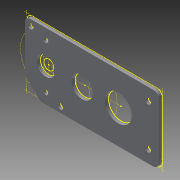
# Autodesk Inventor part: Granny Gearbox Input Plate Routing Template
Saved by Autodesk Inventor 2015 (Build 190159000, 159)
## iProperties
Created: 2016-02-25
Part Number: Granny Gearbox Input Plate Routing Template
Material: Generic
Document SubType Name: Modeling
Designer: sethbattis
Density: 1 g/cm^3
Appearance: Default
Author: sethbattis
Autodesk Inventor part; units mm, degrees
ref_plane "YZ Plane" through (0, 0, 0) normal (1, 0, 0) x (0, 1, 0)
ref_plane "XZ Plane" through (0, 0, 0) normal (0, 1, 0) x (-1, 0, 0)
ref_plane "XY Plane" through (0, 0, 0) normal (0, 0, 1) x (1, 0, 0)
derived "Granny Gearbox Input Plate.ipt"
feature "Solid1::Granny Gearbox Input Plate.ipt" [suppressed]
sketch "Shaft Alignment" plane through (0, 0, 0) normal (0, 0, 1) x (1, 0, 0)
  line L0 (-40.7035, -5.5985) -> (-0.0001, -11.1125) construction
  line L1 (-35.1409, -0.031) -> (-35.1353, -6.3528) construction
  line L2 (-11.1125, -0.0098) -> (-11.104, -9.6083) construction
  line L3 (0, 11.1125) -> (43.74, 13.9583) construction
  line L4 (-40.7035, -5.5985) -> (-46.2661, -5.5985) construction
  line L5 (-40.7035, -19.8733) -> (-46.2661, -19.8733) construction
  line L6 (-40.7035, 19.8015) -> (-46.2661, 19.8015) construction
  line L7 (-40.7035, 5.5267) -> (-46.2661, 5.5267) construction
  line L8 (-46.2661, 25.3641) -> (-46.2661, -25.4359) construction
  line L9 (-40.7035, 25.3641) -> (-40.7035, -25.4359) construction
  line L10 (-40.7035, -0.0359) -> (0, 0) construction
  line L11 (0, 0) -> (40.6908, 0) construction
  line L12 (11.1125, 0) -> (11.1125, 11.8355) construction
  line L13 (26.4033, 0) -> (26.4033, 12.8304) construction
  circle A0 centre (-40.7035, 25.3641) radius 5.5626
  circle A1 centre (-40.7035, -25.4359) radius 5.5626
  circle A2 centre (40.6908, 0) radius 14.2875
  circle A3 centre (0, 0) radius 11.1125
  circle A4 centre (-40.7035, -0.0359) radius 5.5626
  point P0 (-33.5787, -27.5177)
sketch "New Mounting Holes" plane through (0, 0, 0) normal (0, 0, 1) x (1, 0, 0)
  circle A0 centre (-40.7035, -0.0359) radius 31.75 construction
  circle A1 centre (40.6908, 0) radius 36.195 construction
  circle A2 centre (0, 0) radius 36.195 construction
  line L0 (-57.7242, 30.4609) -> (-55.8383, 30.4609) construction
  line L1 (-57.7242, 30.4609) -> (-57.7242, 28.575) construction
  circle A3 centre (-57.7242, 30.4609) radius 3.175
  circle A4 centre (-24.3812, -30.912) radius 3.175
  line L2 (-65.3633, -38.1) -> (-65.3633, 38.1) construction
  line L3 (87.0367, -38.1) -> (-65.3633, -38.1) construction
  line L4 (87.0367, 38.1) -> (87.0367, -38.1) construction
  line L5 (-65.3633, 38.1) -> (87.0367, 38.1) construction
  line L6 (-55.8383, 38.1) -> (-55.8383, -38.1) construction
  line L7 (-65.3633, 28.575) -> (87.0367, 28.575) construction
  line L8 (-65.3633, -28.575) -> (87.0367, -28.575) construction
  line L9 (77.5117, 38.1) -> (77.5117, -38.1) construction
  circle A5 centre (74.3367, 23.3553) radius 3.175
  circle A6 centre (74.3367, -23.3553) radius 3.175
sketch "Labels" plane through (0, 0, 0) normal (0, 0, 1) x (1, 0, 0)
  circle A0 centre (-40.7035, -0.0359) radius 5.5626
  circle A1 centre (-40.7035, 25.3641) radius 5.5626
  circle A2 centre (-40.7035, -25.4359) radius 5.5626
  circle A3 centre (0, 0) radius 11.1125
  circle A4 centre (40.6908, 0) radius 14.2875
  line L0 (-5.8677, 26.2224) -> (48.5566, 26.2224) construction
  line L1 (48.5566, 26.2224) -> (48.5566, 22.1963) construction
  line L2 (48.5566, 22.1963) -> (-5.8677, 22.1963) construction
  line L3 (-5.8677, 22.1963) -> (-5.8677, 26.2224) construction
sketch "Exterior" plane through (0, 0, 0) normal (0, 0, 1) x (1, 0, 0)
  line L0 (-65.3633, -17.4045) -> (-65.3633, 31.75)
  line L1 (-59.0133, 38.1) -> (80.6867, 38.1)
  line L2 (87.0367, 31.75) -> (87.0367, -31.75)
  line L3 (80.6867, -38.1) -> (-44.6678, -38.1)
  arc A0 (87.0367, 31.75) -> (80.6867, 38.1) centre (80.6867, 31.75) ccw
  arc A1 (80.6867, -38.1) -> (87.0367, -31.75) centre (80.6867, -31.75) ccw
  arc A2 (-59.0133, 38.1) -> (-65.3633, 31.75) centre (-59.0133, 31.75) ccw
  circle A3 centre (-40.7035, -0.0359) radius 31.75 construction
  line L4 (-63.5034, -21.8946) -> (-49.1579, -36.2401)
  line L5 (-65.3633, -38.1) -> (-65.3633, 38.1) construction
  line L6 (87.0367, -38.1) -> (-65.3633, -38.1) construction
  arc A4 (-49.1579, -36.2401) -> (-44.6678, -38.1) centre (-44.6678, -31.75) ccw
  arc A5 (-65.3633, -17.4045) -> (-63.5034, -21.8946) centre (-59.0133, -17.4045) ccw
  point P0 (87.0367, 38.1)
  point P1 (-65.3633, -20.0348)
  point P2 (-47.2981, -38.1)
sketch "Input Labels" plane through (0, 0, 0) normal (0, 0, 1) x (1, 0, 0)
  circle A0 centre (-40.7035, 25.3641) radius 2.667
  circle A1 centre (-40.7035, -0.0359) radius 9.525
  circle A2 centre (-40.7035, -25.4359) radius 2.667
  circle A3 centre (0, 0) radius 11.1125
  line L0 (-5.8677, 22.1963) -> (-5.8677, 26.2224) construction
  line L1 (-5.8677, 26.2224) -> (48.5566, 26.2224) construction
  line L2 (48.5566, 26.2224) -> (48.5566, 22.1963) construction
  line L3 (48.5566, 22.1963) -> (-5.8677, 22.1963) construction
  circle A4 centre (40.6908, 0) radius 14.2875
  line L4 (-5.8677, 26.2224) -> (45.7507, 26.2224) construction
  line L5 (45.7507, 26.2224) -> (45.7507, 22.1963) construction
  line L6 (45.7507, 22.1963) -> (-5.8677, 22.1963) construction
  line L7 (-5.8677, 22.1963) -> (-5.8677, 26.2224) construction
sketch "Sketch6" plane through (0, 0, 0) normal (0, 0, 1) x (1, 0, 0)
  line L0 (-63.5034, -21.8946) -> (-49.1579, -36.2401) projected
  line L1 (87.0367, -38.1) -> (-65.3633, -38.1) construction
  line L2 (87.0367, 38.1) -> (87.0367, -38.1) construction
  circle A0 centre (0, 0) radius 11.1125 projected
  circle A1 centre (40.6908, 0) radius 14.2875 projected
  circle A2 centre (-40.7035, 25.3641) radius 2.667 projected
  circle A3 centre (-40.7035, -0.0359) radius 9.525 projected
  circle A4 centre (-40.7035, -25.4359) radius 2.667 projected
  circle A5 centre (-24.3812, -30.912) radius 3.175 projected
  circle A6 centre (-57.7242, 30.4609) radius 3.175 projected
  circle A7 centre (74.3367, -23.3553) radius 3.175 projected
  line L3 (-58.0057, 37.3062) -> (79.893, 37.3062)
  line L4 (86.243, 30.9562) -> (86.243, -30.9562)
  line L5 (79.893, -37.3062) -> (-44.339, -37.3063)
  line L6 (-65.3633, 38.1) -> (87.0367, 38.1) construction
  line L7 (-65.3633, -38.1) -> (-65.3633, 38.1) construction
  line L8 (-62.4958, -21.7797) -> (-48.8291, -35.4464)
  line L9 (-64.3557, -17.2896) -> (-64.3557, 30.9562)
  circle A8 centre (-40.7035, -0.0359) radius 10.3187
  circle A9 centre (0, 0) radius 11.9062
  circle A10 centre (40.6908, 0) radius 15.0812
  circle A11 centre (0, 0) radius 36.195 construction
  arc A12 (86.243, 30.9562) -> (79.893, 37.3062) centre (79.893, 30.9562) ccw
  arc A13 (-58.0057, 37.3062) -> (-64.3557, 30.9562) centre (-58.0057, 30.9562) ccw
  arc A14 (-64.3557, -17.2896) -> (-62.4958, -21.7797) centre (-58.0057, -17.2896) ccw
  arc A15 (-48.8291, -35.4464) -> (-44.339, -37.3063) centre (-44.339, -30.9563) ccw
  arc A16 (79.893, -37.3062) -> (86.243, -30.9562) centre (79.893, -30.9562) ccw
  circle A17 centre (74.3367, 23.3553) radius 3.175 projected
  dimension "d20" = 0.7937
  dimension "d22" = 0.7937
  dimension "d23" = 0.7937
  dimension "d24" = 0.7937
  dimension "d25" = 19.05
  dimension "d26" = 20.6375
  dimension "d27" = 22.225
  dimension "d28" = 23.8125
  dimension "d29" = 28.575
  dimension "d30" = 30.1625
  dimension "d31" = 6.35
  constraints: 10 end point, 10 point on circle, 10 tangent, 8 centre point, 4 equal radius, 3 coincident, 3 parallel, 1 horizontal, 1 perpendicular
  measures "d20" distance between parallel lines of L3 L6
  measures "d22" distance between parallel lines of L1 L5
  measures "d23" distance between parallel lines of L2 L4
  measures "d24" distance between parallel lines of L0 L8
  measures "d25" diameter of A3
  measures "d26" diameter of A8
  measures "d27" diameter of A0
  measures "d28" diameter of A9
  measures "d29" diameter of A1
  measures "d30" diameter of A10
  measures "d31" radius of A12
extrude "Extrusion2" add sketch "Sketch6" along normal blind 3.175 contours L3 A12 L4 A16 L5 A15 L8 A14 L9 A13
equation "\"d22\" = d20"
equation "\"d23\" = d20"
equation "\"d24\" = d20"
equation "\"d26\" = d25 + 2 * d20"
equation "\"d28\" = d27 + 2 * d20"
equation "\"d30\" = d29 + 2 * d20"
body "Solid1"
